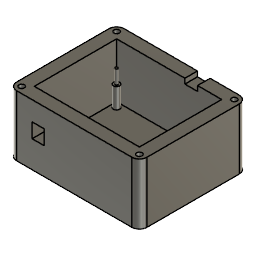
AOILED_CASE (Autodesk Fusion 360 archive; units mm, degrees)
design "BOTTOMPART"
part number: 2026-03-31-16-14-19-935
Autodesk Fusion 360 part; units mm, degrees
sketch "Sketch1" plane through (0, 0, 0) normal (0, 0, 1) x (1, 0, 0)
  line L0 (-45.352, 30.7799) -> (37.648, 30.7799)
  line L1 (37.648, 30.7799) -> (37.648, -34.2201)
  line L2 (37.648, -34.2201) -> (-45.352, -34.2201)
  line L3 (-45.352, -34.2201) -> (-45.352, 30.7799)
  line L4 (-55.352, 40.7799) -> (47.648, 40.7799)
  line L5 (47.648, 40.7799) -> (47.648, -44.2201)
  line L6 (47.648, -44.2201) -> (-55.352, -44.2201)
  line L7 (-55.352, -44.2201) -> (-55.352, 40.7799)
  circle A0 centre (-41.445, 26.7879) radius 2.5
  circle A1 centre (-41.445, 26.7879) radius 1.075
  circle A2 centre (34.648, 26.7879) radius 1.075
  circle A3 centre (34.648, 26.7879) radius 2.5
  circle A4 centre (-41.445, -31.2201) radius 1.075
  circle A5 centre (-41.445, -31.2201) radius 2.5
  circle A6 centre (34.648, -31.2201) radius 1.075
  circle A7 centre (34.648, -31.2201) radius 2.5
  dimension "d1" = 83
  dimension "d2" = 65
  dimension "d3" = 103
  dimension "d4" = 85
  dimension "d5" = 10
  dimension "d6" = 10
  dimension "d7" = 5
  dimension "d8" = 2.15
  dimension "d11" = 2.15
  dimension "d12" = 5
  dimension "d14" = 3
  dimension "d15" = 2.15
  dimension "d16" = 5
  dimension "d17" = 3
  dimension "d19" = 2.15
  dimension "d20" = 5
  dimension "d21" = 3
  dimension "d22" = 3
  dimension "d31" = 76.093
  dimension "d32" = 58.008
  dimension "d33" = 76.093
  dimension "d34" = 58.008
  constraint horizontal L0
  constraint vertical L1
  constraint horizontal L2
  constraint vertical L3
  constraint horizontal L4
  constraint vertical L5
  constraint horizontal L6
  constraint vertical L7
  constraint concentric A0 A1
  constraint concentric A2 A3
  constraint concentric A4 A5
  constraint concentric A6 A7
  measures "d1" distance of L0.start L0.end
  measures "d2" distance of L0.start L2.end
  measures "d3" distance of L4.start L4.end
  measures "d4" distance of L4.start L6.end
  measures "d5" distance of L0 L4
  measures "d6" distance of L3 L7
  measures "d7" diameter of A0
  measures "d8" diameter of A1
  measures "d11" diameter of A2
  measures "d12" diameter of A3
  measures "d14" distance of L1 A2.centre
  measures "d15" diameter of A4
  measures "d16" diameter of A5
  measures "d17" distance of L2 A4.centre
  measures "d19" diameter of A6
  measures "d20" diameter of A7
  measures "d21" distance of L2 A6.centre
  measures "d22" distance of L1 A6.centre
  measures "d31" distance of A4.centre A6.centre
  measures "d32" distance of A2.centre A6.centre
  measures "d33" distance of A0.centre A2.centre
  measures "d34" vertical distance of A0.centre A4.centre
extrude "Extrude1" add sketch "Sketch1" along normal blind 48 contours L4 L5 L6 L7
extrude "Extrude2" add sketch "Sketch1" along normal blind 5 contours L0 L1 L2 L3
extrude "Extrude3" add sketch "Sketch1" along normal blind 21 contours A0 | A3 | A5 | A7
extrude "Extrude4" add sketch "Sketch1" along normal blind 32 contours A1 | A2 | A4 | A6
sketch "Sketch2" plane through (0, -34.2201, 0) normal (0, 1, 0) x (-1, 0, 0)
  line L0 (-37.648, 5) -> (45.352, 5)
  line L1 (45.352, 5) -> (45.352, 48)
  line L2 (45.352, 48) -> (-37.648, 48)
  line L3 (-37.648, 48) -> (-37.648, 5)
  line L4 (27.602, 32.8) -> (37.102, 32.8)
  line L5 (37.102, 32.8) -> (37.102, 21.3)
  line L6 (37.102, 21.3) -> (27.602, 21.3)
  line L7 (27.602, 21.3) -> (27.602, 32.8)
  dimension "d35" = 9.5
  dimension "d36" = 11.5
  dimension "d37" = 16.3
  dimension "d38" = 65.25
  constraint horizontal L4
  constraint vertical L5
  constraint horizontal L6
  constraint vertical L7
  measures "d35" distance of L4.start L4.end
  measures "d36" distance of L4.start L6.end
  measures "d37" distance of L0 L6
  measures "d38" distance of L3 L7
extrude "Extrude5" cut sketch "Sketch2" against normal blind 10 contours L4 L5 L6 L7
sketch "Sketch3" plane through (0, 0, 48) normal (0, 0, 1) x (-1, 0, 0)
  line L0 (-37.648, 34.2201) -> (45.352, 34.2201)
  line L1 (45.352, 34.2201) -> (45.352, -30.7799)
  line L2 (45.352, -30.7799) -> (-37.648, -30.7799)
  line L3 (-37.648, -30.7799) -> (-37.648, 34.2201)
  line L4 (55.352, 44.2201) -> (-47.648, 44.2201)
  line L5 (-47.648, 44.2201) -> (-47.648, -40.7799)
  line L6 (-47.648, -40.7799) -> (55.352, -40.7799)
  line L7 (55.352, -40.7799) -> (55.352, 44.2201)
  line L8 (-18.568, -30.7799) -> (-8.568, -30.7799)
  line L9 (-8.568, -30.7799) -> (-8.568, -40.7799)
  line L10 (-8.568, -40.7799) -> (-18.568, -40.7799)
  line L11 (-18.568, -40.7799) -> (-18.568, -30.7799)
  dimension "d41" = 10
  constraint horizontal L8
  constraint vertical L9
  constraint horizontal L10
  constraint vertical L11
  constraint coincident L2 L8.start
  measures "d41" distance of L8.start L8.end
extrude "Extrude6" cut sketch "Sketch3" against normal blind 4 contours L2 L6 L8 L9 L10 L11
sketch "Sketch4" plane through (0, 0, 48) normal (0, 0, 1) x (-1, 0, 0)
  line L0 (-8.568, -30.7799) -> (-8.568, -40.7799)
  line L1 (-8.568, -40.7799) -> (55.352, -40.7799)
  line L2 (55.352, -40.7799) -> (55.352, 44.2201)
  line L3 (55.352, 44.2201) -> (-47.648, 44.2201)
  line L4 (-47.648, 44.2201) -> (-47.648, -40.7799)
  line L5 (-47.648, -40.7799) -> (-18.568, -40.7799)
  line L6 (-18.568, -40.7799) -> (-18.568, -30.7799)
  line L7 (-18.568, -30.7799) -> (-37.648, -30.7799)
  line L8 (-37.648, -30.7799) -> (-37.648, 34.2201)
  line L9 (-37.648, 34.2201) -> (45.352, 34.2201)
  line L10 (45.352, 34.2201) -> (45.352, -30.7799)
  line L11 (45.352, -30.7799) -> (-8.568, -30.7799)
  circle A0 centre (-42.648, 39.2201) radius 2.15
  circle A1 centre (50.352, 39.2201) radius 2.15
  circle A2 centre (-42.648, -35.7799) radius 2.15
  circle A3 centre (50.352, -35.7799) radius 2.15
  dimension "d44" = 4.3
  dimension "d45" = 5
  dimension "d46" = 5
  dimension "d47" = 4.3
  dimension "d48" = 5
  dimension "d49" = 5
  dimension "d50" = 4.3
  dimension "d51" = 5
  dimension "d52" = 5
  dimension "d53" = 4.3
  dimension "d54" = 5
  dimension "d55" = 5
  measures "d44" diameter of A0
  measures "d45" distance of L3 A0.centre
  measures "d46" distance of L4 A0.centre
  measures "d47" diameter of A1
  measures "d48" distance of L2 A1.centre
  measures "d49" distance of L3 A1.centre
  measures "d50" diameter of A2
  measures "d51" distance of L4 A2.centre
  measures "d52" distance of L5 A2.centre
  measures "d53" diameter of A3
  measures "d54" distance of L2 A3.centre
  measures "d55" distance of L1 A3.centre
extrude "Extrude7" cut sketch "Sketch4" against normal blind 30 contours A0 | A1 | A2 | A3
fillet "Fillet1" radius 6 4 edges at (-55.352, -44.2201, 24) (-55.352, 40.7799, 24) (47.648, -44.2201, 24) (47.648, 40.7799, 24)
